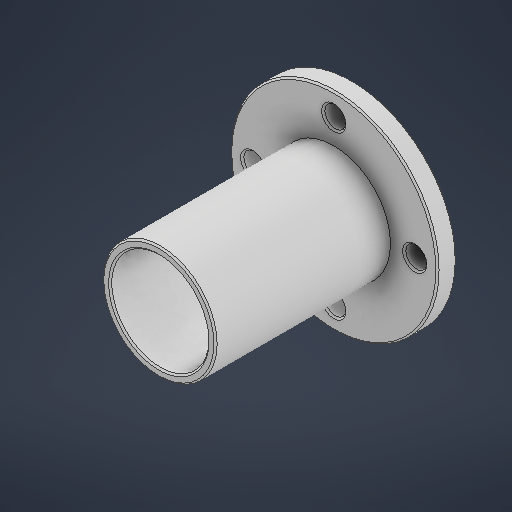
# Autodesk Inventor part: Cylinder
Saved by Autodesk Inventor 2025.4 (Build 294407000, 407)
## iProperties
Created: 2026-05-29
Part Number: Cylinder
Material: Generic
Document SubType Name: Modeling
Designer: VuQuan
Density: 1 g/cm^3
Appearance: Default
Author: VuQuan
Autodesk Inventor part; units mm, degrees
ref_plane "YZ Plane" through (0, 0, 0) normal (1, 0, 0) x (0, 1, 0)
ref_plane "XZ Plane" through (0, 0, 0) normal (0, 1, 0) x (-1, 0, 0)
ref_plane "XY Plane" through (0, 0, 0) normal (0, 0, 1) x (1, 0, 0)
sketch "Sketch1" plane through (0, 0, 0) normal (0, 0, 1) x (1, 0, 0)
  circle A0 centre (0, 0) radius 32
  circle A1 centre (0, 0) radius 20
  circle A2 centre (0, 0) radius 17.5
  circle A3 centre (0, 0) radius 15
  circle A4 centre (0, 25) radius 3.25
  circle A5 centre (-25, 0) radius 3.25
  circle A6 centre (0, -25) radius 3.25
  circle A7 centre (25, 0) radius 3.25
  dimension "d0" = 64
  dimension "d1" = 40
  dimension "d2" = 35
  dimension "d3" = 30
  dimension "d4" = 6.5
  dimension "d5" = 25
  dimension "d8" = 360
  constraints: 8 centre point, 4 coincident, 1 vertical alignment, 9 other
  measures "d0" diameter of A0
  measures "d1" diameter of A1
  measures "d2" diameter of A2
  measures "d3" diameter of A3
  measures "d4" diameter of A4
  measures "d5" distance of A4.centre point (0, 0)
extrude "Extrusion1" add sketch "Sketch1" along normal blind 6 contours A0 | A1 | A2
extrude "Extrusion2" add sketch "Sketch1" along normal blind 60 contours A2
extrude "Extrusion3" cut sketch "Sketch1" along normal blind 2.3 contours A1 | A2 | A3
chamfer "Chamfer1" distance 0.5 angle 45 13 edges at (-32, 0, 0) (-32, 0, 6) (-17.5, 0, 60) (-15, 0, 60) (-15, 0, 2.3) (-3.25, -25, 0) (-28.25, 0, 0) (-3.25, 25, 0) (21.75, 0, 0) (-28.25, 0, 6) (-3.25, -25, 6) (21.75, 0, 6) (-3.25, 25, 6)
body "Solid1"
